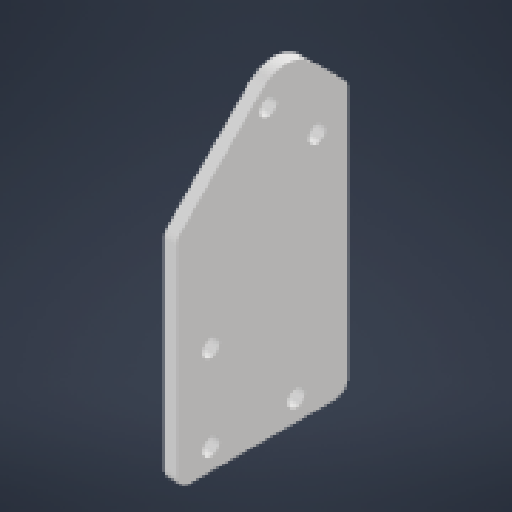
# Autodesk Inventor part: Arm_Servo_Holder
Saved by Autodesk Inventor 2026.1 (Build 301233020, 233B)
## iProperties
Created: 2025-10-29
Part Number: Arm_Servo_Holder
Material: Generic
Document SubType Name: Modeling
Designer: Garfieldcmix
Density: 1 g/cm^3
Appearance: Default
Author: Garfieldcmix
Autodesk Inventor part; units mm, degrees
ref_plane "YZ Plane" through (0, 0, 0) normal (1, 0, 0) x (0, 1, 0)
ref_plane "XZ Plane" through (0, 0, 0) normal (0, 1, 0) x (-1, 0, 0)
ref_plane "XY Plane" through (0, 0, 0) normal (0, 0, 1) x (1, 0, 0)
sketch "Sketch1" plane through (0, 0, 0) normal (1, 0, 0) x (0, 1, 0)
  line L0 (0, 0) -> (0, 40)
  line L1 (0, 40) -> (82, 40) construction
  line L2 (82, 40) -> (43, 0) construction
  line L3 (43, 0) -> (0, 0)
  line L4 (85.0695, 14.499) -> (70.933, 0)
  line L5 (70.933, 0) -> (43, 0)
  line L6 (85.0695, 14.499) -> (70.7495, 28.461)
  circle A0 centre (75.1171, 18.616) radius 2
  circle A1 centre (63.9475, 7.16) radius 2
  line L7 (77.9095, 21.48) -> (56.9665, 0) construction
  circle A2 centre (25, 32) radius 2
  circle A3 centre (5, 32) radius 2
  circle A4 centre (5, 12) radius 2
  line L8 (25, 32) -> (5, 32) construction
  line L9 (5, 32) -> (5, 12) construction
  line L10 (70.7495, 28.461) -> (58.9146, 40)
  line L11 (0, 40) -> (58.9146, 40)
  dimension "d0" = 43
  dimension "d1" = 39
  dimension "d2" = 40
  dimension "d4" = 4
  dimension "d5" = 16
  dimension "d6" = 4
  dimension "d7" = 4
  dimension "d8" = 20
  dimension "d9" = 20
  dimension "d10" = 8
  dimension "d11" = 5
  dimension "d16" = 20
  dimension "d17" = 10
  constraints: 24 end point, 5 centre point, 4 point on line, 3 equal radius, 3 horizontal, 2 collinear, 2 midpoint, 2 perpendicular, 2 vertical, 1 parallel
  measures "d0" distance of L2.end L0.start
  measures "d1" horizontal distance of L1.end L2.end
  measures "d2" distance of L0.start L0.end
  measures "d4" diameter of A0
  measures "d5" distance of A1.centre A0.centre
  measures "d6" distance from line of L6 A0.centre
  measures "d7" diameter of A2
  measures "d8" distance of L8.start L8.end
  measures "d9" distance of L8.end L9.end
  measures "d10" distance from line of L1 L8.end
  measures "d11" distance from line of L0 L8.end
  measures "d16" distance between parallel lines of L2 L4
  measures "d17" distance of L7.end A1.centre
extrude "Extrusion1" add sketch "Sketch1" along normal blind 3
fillet "Fillet1" radius 3 4 edges at (1.5, 58.9146, 40) (1.5, 70.933, 0) (1.5, 0, 40) (1.5, 0, 0)
fillet "Fillet2" radius 8 1 edges at (1.5, 85.0695, 14.499)
body "Solid1"
